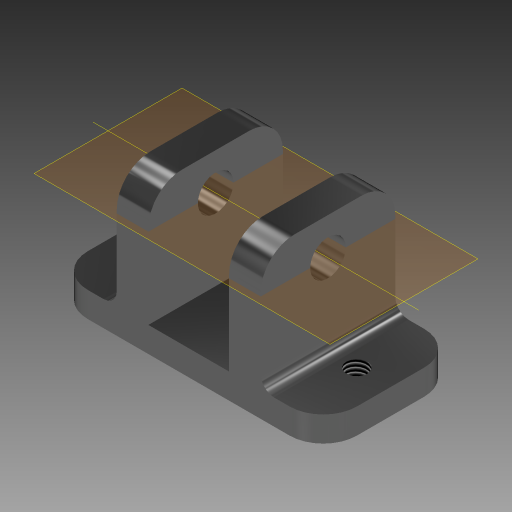
# Autodesk Inventor part: TTB 4mm Dyneema Cable Pulley Bracket (ELEV-PULLEY-001)
Saved by Autodesk Inventor 2023 (Build 270158000, 158)
## iProperties
Created: 2022-11-17
Part Number: TTB 4mm Dyneema Cable Pulley Bracket (ELEV-PULLEY-001)
Material: Aluminum 6061
Document SubType Name: Modeling
Designer: Max Boord
Mass: 32.5106 g
Surface Area: 59.6921 cm^2
Volume: 12.041 cm^3
Density: 2.7 g/cm^3
Appearance: Glazed - Black
Author: Max Boord
Autodesk Inventor part; units mm, degrees
ref_plane "YZ Plane" through (0, 0, 0) normal (1, 0, 0) x (0, 1, 0)
ref_plane "XY Plane" through (0, 0, 0) normal (0, 0, 1) x (1, 0, 0)
sketch "Sketch1" plane through (0, 0, 0) normal (0, 0, 1) x (1, 0, 0)
  line L0 (-25.4, 4.7625) -> (-25.4, 0)
  line L1 (-25.4, 0) -> (25.4, 0)
  line L2 (25.4, 0) -> (25.4, 4.7625)
  line L3 (25.4, 4.7625) -> (-25.4, 0) construction
  line L4 (-25.4, 4.7625) -> (25.4, 0) construction
  line L5 (-7.62, 4.7625) -> (-7.62, 26.9875)
  line L6 (-7.62, 26.9875) -> (-13.589, 26.9875)
  line L7 (-13.589, 26.9875) -> (-13.589, 7.3025)
  line L8 (13.589, 7.3025) -> (13.589, 26.9875)
  line L9 (13.589, 26.9875) -> (7.62, 26.9875)
  line L10 (7.62, 26.9875) -> (7.62, 4.7625)
  line L11 (0, 4.7625) -> (0, 30.1851) construction
  line L12 (-16.129, 4.7625) -> (-25.4, 4.7625)
  line L13 (25.4, 4.7625) -> (16.129, 4.7625)
  line L14 (7.62, 4.7625) -> (-7.62, 4.7625)
  arc A0 (-16.129, 4.7625) -> (-13.589, 7.3025) centre (-16.129, 7.3025) ccw
  arc A1 (13.589, 7.3025) -> (16.129, 4.7625) centre (16.129, 7.3025) ccw
  point P0 (0, 0)
  point P1 (0, 2.3812)
  point P2 (0, 0)
  dimension "d0" = 26.9875
  dimension "d2" = 50.8
  dimension "d3" = 5.969
  dimension "d4" = 15.24
  dimension "d5" = 2.54
  dimension "d6" = 4.7625
  constraints: 30 end point, 6 parallel, 5 midpoint, 4 point on circle, 4 tangent, 3 equal length, 3 horizontal, 3 perpendicular, 2 centre point, 2 horizontal alignment, 1 coincident, 1 equal radius, 1 vertical, 1 vertical alignment, 1 other
  measures "d0" distance between parallel lines of L1 L6
  measures "d2" distance between parallel lines of L0 L2
  measures "d3" distance of L5.end L6.end
  measures "d4" distance between parallel lines of L10 L5
  measures "d5" radius of A0
  measures "d6" distance between parallel lines of L1 L12
extrude "Extrusion1" add sketch "Sketch1" along normal mid plane 25.4
fillet "Fillet1" radius 6.35 8 edges at (-10.6045, 26.9875, 12.7) (10.6045, 26.9875, 12.7) (-10.6045, 26.9875, -12.7) (10.6045, 26.9875, -12.7) (25.4, 2.3813, 12.7) (25.4, 2.3813, -12.7) (-25.4, 2.3813, 12.7) (-25.4, 2.3813, -12.7)
sketch "Sketch2" plane through (-13.589, 7.3025, -12.7) normal (-1, 0, 0) x (0, 0, 1)
  circle A0 centre (12.7, 12.7) radius 3.3655
  line L0 (6.35, -7.3025) -> (19.05, -7.3025) projected
  point P0 (12.7, -7.3025)
  point P1 (25.4, -2.54)
  point P2 (12.7, -7.3025)
  dimension "d10" = 6.731
  dimension "d11" = 15.24
  constraints: 1 centre point, 1 midpoint, 1 vertical alignment
  measures "d10" diameter of A0
  measures "d11" vertical distance of point (25.4, -2.54) A0.centre
extrude "Extrusion2" cut sketch "Sketch2" against normal through all
sketch "Sketch3" plane through (-19.05, 0, -12.7) normal (0, -1, 0) x (1, 0, 0)
  line L0 (0, 12.7) -> (38.1, 12.7) construction
  circle A0 centre (0, 12.7) radius 2.0193
  circle A1 centre (38.1, 12.7) radius 2.0193
  point P0 (19.05, 12.7)
  point P1 (19.05, 12.7)
  dimension "d14" = 4.0386
  dimension "d15" = 38.1
  constraints: 3 coincident, 2 centre point, 2 end point, 1 equal radius, 1 horizontal, 1 midpoint
  measures "d14" diameter of A0
  measures "d15" distance of L0.start L0.end
hole "Hole1" at (-19.05, 0, 0) at (19.05, 0, 0) direction (0, 1, 0) diameter 3.9624 end through all thread size "10-32 UNF" class "2B" standard "ANSI Unified Screw Threads"
ref_plane "Work Plane1" through (-13.589, 20.0025, 0) normal (0, 1, 0) x (1, 0, 0)
body "Solid1"
